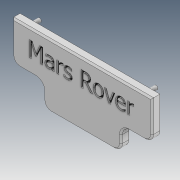
# Autodesk Inventor part: tampa parte de traz mars
Saved by Autodesk Inventor 2021 (Build 250183000, 183)
## iProperties
Created: 2020-11-19
Part Number: tampa parte de traz mars
Material: Genérico
Document SubType Name: Modeling
Designer: evert
Density: 1 g/cm^3
Appearance: Padrão
Author: evert
Autodesk Inventor part; units mm, degrees
ref_plane "YZ Plane" through (0, 0, 0) normal (1, 0, 0) x (0, 1, 0)
ref_plane "XZ Plane" through (0, 0, 0) normal (0, 1, 0) x (-1, 0, 0)
ref_plane "XY Plane" through (0, 0, 0) normal (0, 0, 1) x (1, 0, 0)
sketch "Esboço1" plane through (0, 0, 0) normal (0, 0, 1) x (1, 0, 0)
  line L0 (0, 0) -> (180, 0)
  line L1 (180, 0) -> (180, -50.8)
  line L2 (180, -50.8) -> (0, -50.8)
  line L3 (0, -50.8) -> (0, 0)
  line L4 (0, -50.8) -> (40, -50.8)
  line L5 (40, -50.8) -> (40, -80.8)
  line L6 (40, -80.8) -> (140, -80.8)
  line L7 (140, -80.8) -> (140, -50.8)
  dimension "d0" = 180
  dimension "d1" = 50.8
  dimension "d2" = 40
  dimension "d3" = 30
  dimension "d4" = 100
  constraints: 16 end point, 5 perpendicular, 2 point on line, 1 horizontal, 1 vertical
  measures "d0" distance of L0.start L0.end
  measures "d1" distance of L0.end L1.end
  measures "d2" distance of L2.end L4.end
  measures "d3" distance of L4.end L5.end
  measures "d4" distance of L5.end L6.end
extrude "Extrusão1" add sketch "Esboço1" along normal blind 10
sketch "Esboço3" plane through (0, 0, 0) normal (0, 0, -1) x (-1, 0, 0)
  line L0 (-40, -50.8) -> (-40, -80.8) projected
  line L1 (-40, -80.8) -> (0, -80.8) projected
  line L2 (-40, -50.8) -> (0, -50.8)
  line L3 (0, -50.8) -> (0, -80.8)
  line L4 (0, -80.8) -> (-40, -80.8)
  line L5 (-40, -80.8) -> (-40, -50.8)
  line L6 (-140, -50.8) -> (-180, -50.8) projected
  line L7 (-180, -40.4) -> (-180, -80.8) projected
  line L8 (-140, -50.8) -> (-180, -50.8)
  line L9 (-180, -50.8) -> (-180, -80.8)
  line L10 (-180, -80.8) -> (-140, -80.8)
  line L11 (-140, -80.8) -> (-140, -50.8)
  point P0 (0, 0)
  constraints: 16 end point, 4 parallel, 2 horizontal, 2 perpendicular
extrude "Extrusão3" cut sketch "Esboço3" against normal blind 180
sketch "Esboço4" plane through (0, 0, 0) normal (0, 0, -1) x (-1, 0, 0)
  line L0 (-180, 0) -> (0, 0) projected
  line L1 (0, 0) -> (-15, 0)
  line L2 (-15, 0) -> (-15, -5)
  line L3 (0, -8.08) -> (-180, -8.08) projected
  circle A0 centre (-15, -5) radius 2.5
  line L4 (0, -50.8) -> (0, -40.4) projected
  line L5 (0, -50.8) -> (-15, -50.8)
  line L6 (-15, -50.8) -> (-15, -35.8)
  circle A1 centre (-15, -35.8) radius 2.5
  line L7 (-40, -80.8) -> (-140, -80.8) projected
  line L8 (-40, -80.8) -> (-55, -80.8)
  line L9 (-55, -80.8) -> (-55, -65.8)
  circle A2 centre (-55, -65.8) radius 2.5
  line L10 (-140, -80.8) -> (-140, -50.8) projected
  line L11 (-140, -80.8) -> (-125, -80.8)
  line L12 (-125, -80.8) -> (-125, -65.8)
  circle A3 centre (-125, -65.8) radius 2.5
  line L13 (-140, -50.8) -> (-180, -50.8) projected
  line L14 (-180, -50.8) -> (-165, -50.8)
  line L15 (-165, -50.8) -> (-165, -35.8)
  circle A4 centre (-165, -35.8) radius 2.5
  line L16 (-180, 0) -> (-165, 0)
  line L17 (-165, 0) -> (-165, -5)
  circle A5 centre (-165, -5) radius 2.5
  dimension "d13" = 15
  dimension "d14" = 5
  dimension "d15" = 15
  dimension "d16" = 5
  dimension "d17" = 15
  dimension "d18" = 15
  dimension "d19" = 5
  dimension "d20" = 15
  dimension "d21" = 15
  dimension "d22" = 15
  constraints: 24 end point, 6 centre point, 6 coincident, 5 point on line, 4 perpendicular, 3 vertical
  measures "d13" distance of L0.end L1.end
  measures "d14" distance of L1.end L2.end
  measures "d15" distance of L5.end L6.end
  measures "d16" diameter of A1
  measures "d17" distance of L7.start L8.end
  measures "d18" distance of L8.end L9.end
  measures "d19" diameter of A2
  measures "d20" distance of L7.end L11.end
  measures "d21" distance of L11.end L12.end
  measures "d22" distance of L13.end L14.end
extrude "Extrusão4" add sketch "Esboço4" along normal blind 10
fillet "Arredondamento2" radius 10 6 edges at (140, -50.8, 5) (180, -50.8, 5) (140, -80.8, 5) (40, -80.8, 5) (40, -50.8, 5) (0, -50.8, 5)
chamfer "Chanfro1" distance 2 angle 45 6 edges at (90, 0, 10) (180, -20.4, 10) (0, -20.4, 10) (42.9289, -77.8711, 10) (90, -80.8, 10) (137.0711, -77.8711, 10)
sketch "Esboço7" plane through (0, 0, 10) normal (0, 0, 1) x (1, 0, 0)
  line L0 (20, -13.0888) -> (160, -13.0888) construction
  line L1 (160, -13.0888) -> (160, -33.5102) construction
  line L2 (160, -33.5102) -> (20, -33.5102) construction
  line L3 (20, -33.5102) -> (20, -13.0888) construction
  line L4 (2, -40.8) -> (2, -2) projected
  line L5 (178, -2) -> (178, -40.8) projected
  line L6 (39.1734, -33.0888) -> (36.5154, -33.0888)
  line L7 (36.5154, -33.0888) -> (36.5154, -15.8603)
  line L8 (36.5154, -15.8603) -> (31.2966, -27.5783)
  line L9 (31.2966, -27.5783) -> (29.6759, -27.5783)
  line L10 (29.6759, -27.5783) -> (24.5057, -15.8603)
  line L11 (24.5057, -15.8603) -> (24.5057, -33.0888)
  line L12 (24.5057, -33.0888) -> (22.0259, -33.0888)
  line L13 (22.0259, -33.0888) -> (22.0259, -13.0888)
  line L14 (22.0259, -13.0888) -> (25.6564, -13.0888)
  line L15 (25.6564, -13.0888) -> (30.6483, -24.2234)
  line L16 (30.6483, -24.2234) -> (35.4781, -13.0888)
  line L17 (35.4781, -13.0888) -> (39.1734, -13.0888)
  line L18 (39.1734, -13.0888) -> (39.1734, -33.0888)
  spline S0 degree 2 poles (51.3938, -31.5005) (51.0859, -31.7274) (50.0486, -32.5378) (49.5624, -32.7809) knots 0 0 0 1 2 2 2
  spline S1 degree 2 poles (49.5624, -32.7809) (48.8979, -33.1375) (47.6499, -33.5102) (46.5154, -33.5102) knots 0 0 0 1 2 2 2
  spline S2 degree 2 poles (46.5154, -33.5102) (45.5916, -33.5102) (43.9222, -32.8133) (43.2901, -32.1812) knots 0 0 0 1 2 2 2
  spline S3 degree 2 poles (43.2901, -32.1812) (42.6904, -31.5653) (41.9611, -29.7501) (41.9611, -28.7452) knots 0 0 0 1 2 2 2
  spline S4 degree 2 poles (41.9611, -28.7452) (41.9611, -27.1893) (43.2739, -24.9851) (44.7002, -24.353) knots 0 0 0 1 2 2 2
  spline S5 degree 2 poles (44.7002, -24.353) (45.9643, -23.7696) (49.4003, -23.332) (51.3938, -23.2185) knots 0 0 0 1 2 2 2
  line L19 (51.3938, -23.2185) -> (51.3938, -22.7323)
  spline S6 degree 2 poles (51.3938, -22.7323) (51.3938, -21.8571) (50.859, -20.7712) (50.3728, -20.4632) knots 0 0 0 1 2 2 2
  spline S7 degree 2 poles (50.3728, -20.4632) (49.8865, -20.1553) (48.4927, -19.9608) (47.7472, -19.9608) knots 0 0 0 1 2 2 2
  spline S8 degree 2 poles (47.7472, -19.9608) (46.872, -19.9608) (44.5057, -20.4794) (43.3225, -20.9819) knots 0 0 0 1 2 2 2
  line L20 (43.3225, -20.9819) -> (43.1767, -20.9819)
  line L21 (43.1767, -20.9819) -> (43.1767, -18.4049)
  spline S9 degree 2 poles (43.1767, -18.4049) (43.8736, -18.2104) (46.483, -17.7242) (47.7634, -17.7242) knots 0 0 0 1 2 2 2
  spline S10 degree 2 poles (47.7634, -17.7242) (49.3193, -17.7242) (51.4425, -18.2104) (52.2853, -18.8425) knots 0 0 0 1 2 2 2
  spline S11 degree 2 poles (52.2853, -18.8425) (53.1118, -19.4584) (53.9222, -21.4195) (53.9222, -22.8295) knots 0 0 0 1 2 2 2
  line L22 (53.9222, -22.8295) -> (53.9222, -33.0888)
  line L23 (53.9222, -33.0888) -> (51.3938, -33.0888)
  line L24 (51.3938, -33.0888) -> (51.3938, -31.5005)
  line L25 (51.3938, -29.3935) -> (51.3938, -25.2282)
  spline S12 degree 2 poles (51.3938, -25.2282) (50.4862, -25.3093) (47.7472, -25.5848) (46.8882, -25.8441) knots 0 0 0 1 2 2 2
  spline S13 degree 2 poles (46.8882, -25.8441) (45.8833, -26.1521) (44.5705, -27.4324) (44.5705, -28.567) knots 0 0 0 1 2 2 2
  spline S14 degree 2 poles (44.5705, -28.567) (44.5705, -29.8636) (46.0292, -31.1764) (47.423, -31.1764) knots 0 0 0 1 2 2 2
  spline S15 degree 2 poles (47.423, -31.1764) (48.6062, -31.1764) (50.5511, -30.1553) (51.3938, -29.3935) knots 0 0 0 1 2 2 2
  line L26 (65.4295, -20.7874) -> (65.2998, -20.7874)
  spline S16 degree 2 poles (65.2998, -20.7874) (65.0081, -20.7063) (64.376, -20.6739) (63.9384, -20.6739) knots 0 0 0 1 2 2 2
  spline S17 degree 2 poles (63.9384, -20.6739) (62.9173, -20.6739) (60.9076, -21.5653) (60, -22.4405) knots 0 0 0 1 2 2 2
  line L27 (60, -22.4405) -> (60, -33.0888)
  line L28 (60, -33.0888) -> (57.4716, -33.0888)
  line L29 (57.4716, -33.0888) -> (57.4716, -18.0807)
  line L30 (57.4716, -18.0807) -> (60, -18.0807)
  line L31 (60, -18.0807) -> (60, -20.3174)
  spline S18 degree 2 poles (60, -20.3174) (61.3776, -19.0856) (63.436, -18.0807) (64.4084, -18.0807) knots 0 0 0 1 2 2 2
  spline S19 degree 2 poles (64.4084, -18.0807) (64.7974, -18.0807) (65.1864, -18.1132) (65.4295, -18.1618) knots 0 0 0 1 2 2 2
  line L32 (65.4295, -18.1618) -> (65.4295, -20.7874)
  spline S20 degree 2 poles (71.4425, -33.4454) (69.9352, -33.4454) (67.3258, -32.635) (66.4668, -32.1812) knots 0 0 0 1 2 2 2
  line L33 (66.4668, -32.1812) -> (66.4668, -29.3449)
  line L34 (66.4668, -29.3449) -> (66.5964, -29.3449)
  spline S21 degree 2 poles (66.5964, -29.3449) (66.9206, -29.6042) (67.7958, -30.2201) (68.5251, -30.5605) knots 0 0 0 1 2 2 2
  spline S22 degree 2 poles (68.5251, -30.5605) (69.1572, -30.8684) (70.7131, -31.3222) (71.5397, -31.3222) knots 0 0 0 1 2 2 2
  spline S23 degree 2 poles (71.5397, -31.3222) (72.1394, -31.3222) (73.517, -31.0467) (73.8412, -30.8198) knots 0 0 0 1 2 2 2
  spline S24 degree 2 poles (73.8412, -30.8198) (74.3112, -30.5119) (74.7326, -29.8149) (74.7326, -29.1018) knots 0 0 0 1 2 2 2
  spline S25 degree 2 poles (74.7326, -29.1018) (74.7326, -28.2104) (73.7601, -27.2866) (72.5122, -26.9786) knots 0 0 0 1 2 2 2
  spline S26 degree 2 poles (72.5122, -26.9786) (72.0259, -26.8652) (70.47, -26.541) (69.8055, -26.3627) knots 0 0 0 1 2 2 2
  spline S27 degree 2 poles (69.8055, -26.3627) (68.0875, -25.8603) (66.5316, -23.7858) (66.5316, -22.3109) knots 0 0 0 1 2 2 2
  spline S28 degree 2 poles (66.5316, -22.3109) (66.5316, -20.2687) (69.5948, -17.7242) (72.1232, -17.7242) knots 0 0 0 1 2 2 2
  spline S29 degree 2 poles (72.1232, -17.7242) (73.3712, -17.7242) (75.8995, -18.3401) (76.7585, -18.8101) knots 0 0 0 1 2 2 2
  line L35 (76.7585, -18.8101) -> (76.7585, -21.5167)
  line L36 (76.7585, -21.5167) -> (76.6288, -21.5167)
  spline S30 degree 2 poles (76.6288, -21.5167) (75.6564, -20.7388) (73.2901, -19.8474) (72.0746, -19.8474) knots 0 0 0 1 2 2 2
  spline S31 degree 2 poles (72.0746, -19.8474) (70.8266, -19.8474) (69.1086, -20.9008) (69.1086, -21.9543) knots 0 0 0 1 2 2 2
  spline S32 degree 2 poles (69.1086, -21.9543) (69.1086, -22.9106) (70.1297, -23.8344) (71.2642, -24.1261) knots 0 0 0 1 2 2 2
  spline S33 degree 2 poles (71.2642, -24.1261) (71.8152, -24.272) (73.2091, -24.5637) (73.9708, -24.742) knots 0 0 0 1 2 2 2
  spline S34 degree 2 poles (73.9708, -24.742) (75.624, -25.1634) (77.3096, -27.0921) (77.3096, -28.7615) knots 0 0 0 1 2 2 2
  spline S35 degree 2 poles (77.3096, -28.7615) (77.3096, -29.7339) (76.5478, -31.4519) (75.8023, -32.084) knots 0 0 0 1 2 2 2
  spline S36 degree 2 poles (75.8023, -32.084) (75.0081, -32.7485) (72.9822, -33.4454) (71.4425, -33.4454) knots 0 0 0 1 2 2 2
  line L37 (103.9222, -33.0888) -> (100.47, -33.0888)
  line L38 (100.47, -33.0888) -> (94.1491, -25.131)
  line L39 (94.1491, -25.131) -> (91.1021, -25.131)
  line L40 (91.1021, -25.131) -> (91.1021, -33.0888)
  line L41 (91.1021, -33.0888) -> (88.4441, -33.0888)
  line L42 (88.4441, -33.0888) -> (88.4441, -13.0888)
  line L43 (88.4441, -13.0888) -> (93.5981, -13.0888)
  spline S37 degree 2 poles (93.5981, -13.0888) (95.316, -13.0888) (97.6337, -13.4616) (98.6872, -14.1423) knots 0 0 0 1 2 2 2
  spline S38 degree 2 poles (98.6872, -14.1423) (99.7407, -14.823) (100.9562, -16.9462) (100.9562, -18.5183) knots 0 0 0 1 2 2 2
  spline S39 degree 2 poles (100.9562, -18.5183) (100.9562, -20.7063) (98.7196, -23.6723) (96.8071, -24.3854) knots 0 0 0 1 2 2 2
  line L44 (96.8071, -24.3854) -> (103.9222, -33.0888)
  spline S40 degree 2 poles (98.1848, -18.729) (98.1848, -17.8538) (97.5689, -16.5086) (96.9206, -16.071) knots 0 0 0 1 2 2 2
  spline S41 degree 2 poles (96.9206, -16.071) (96.3533, -15.6982) (94.846, -15.3903) (93.7439, -15.3903) knots 0 0 0 1 2 2 2
  line L45 (93.7439, -15.3903) -> (91.1021, -15.3903)
  line L46 (91.1021, -15.3903) -> (91.1021, -22.9106)
  line L47 (91.1021, -22.9106) -> (93.436, -22.9106)
  spline S42 degree 2 poles (93.436, -22.9106) (94.5867, -22.9106) (96.4182, -22.5054) (97.0502, -21.8733) knots 0 0 0 1 2 2 2
  spline S43 degree 2 poles (97.0502, -21.8733) (97.6337, -21.3222) (98.1848, -19.7663) (98.1848, -18.729) knots 0 0 0 1 2 2 2
  spline S44 degree 2 poles (117.6499, -25.5848) (117.6499, -29.3773) (114.0032, -33.5102) (110.9562, -33.5102) knots 0 0 0 1 2 2 2
  spline S45 degree 2 poles (110.9562, -33.5102) (107.8282, -33.5102) (104.2464, -29.2477) (104.2464, -25.5848) knots 0 0 0 1 2 2 2
  spline S46 degree 2 poles (104.2464, -25.5848) (104.2464, -21.8247) (107.9417, -17.6593) (110.9562, -17.6593) knots 0 0 0 1 2 2 2
  spline S47 degree 2 poles (110.9562, -17.6593) (114.0032, -17.6593) (117.6499, -21.8085) (117.6499, -25.5848) knots 0 0 0 1 2 2 2
  spline S48 degree 2 poles (115.0405, -25.5848) (115.0405, -22.6674) (112.9173, -19.8311) (110.9562, -19.8311) knots 0 0 0 1 2 2 2
  spline S49 degree 2 poles (110.9562, -19.8311) (108.9951, -19.8311) (106.8558, -22.6674) (106.8558, -25.5848) knots 0 0 0 1 2 2 2
  spline S50 degree 2 poles (106.8558, -25.5848) (106.8558, -28.4211) (108.9951, -31.3384) (110.9562, -31.3384) knots 0 0 0 1 2 2 2
  spline S51 degree 2 poles (110.9562, -31.3384) (112.9011, -31.3384) (115.0405, -28.4697) (115.0405, -25.5848) knots 0 0 0 1 2 2 2
  line L48 (132.0259, -18.0807) -> (126.3695, -33.0888)
  line L49 (126.3695, -33.0888) -> (124.1005, -33.0888)
  line L50 (124.1005, -33.0888) -> (118.4927, -18.0807)
  line L51 (118.4927, -18.0807) -> (121.2318, -18.0807)
  line L52 (121.2318, -18.0807) -> (125.3323, -29.6367)
  line L53 (125.3323, -29.6367) -> (129.4003, -18.0807)
  line L54 (129.4003, -18.0807) -> (132.0259, -18.0807)
  spline S52 degree 2 poles (140.4538, -33.4292) (136.8558, -33.4292) (132.9011, -29.3935) (132.9011, -25.6658) knots 0 0 0 1 2 2 2
  spline S53 degree 2 poles (132.9011, -25.6658) (132.9011, -22.0029) (136.7423, -17.6593) (139.8379, -17.6593) knots 0 0 0 1 2 2 2
  spline S54 degree 2 poles (139.8379, -17.6593) (141.2318, -17.6593) (143.3874, -18.4697) (144.1815, -19.3287) knots 0 0 0 1 2 2 2
  spline S55 degree 2 poles (144.1815, -19.3287) (144.9919, -20.1877) (145.8509, -22.6674) (145.8509, -24.4665) knots 0 0 0 1 2 2 2
  line L55 (145.8509, -24.4665) -> (145.8509, -25.8441)
  line L56 (145.8509, -25.8441) -> (135.4619, -25.8441)
  spline S56 degree 2 poles (135.4619, -25.8441) (135.4619, -28.4535) (138.0875, -31.225) (140.4214, -31.225) knots 0 0 0 1 2 2 2
  spline S57 degree 2 poles (140.4214, -31.225) (141.248, -31.225) (142.8525, -30.8522) (143.5008, -30.5605) knots 0 0 0 1 2 2 2
  spline S58 degree 2 poles (143.5008, -30.5605) (144.1815, -30.2363) (145.1216, -29.6691) (145.4295, -29.4097) knots 0 0 0 1 2 2 2
  line L57 (145.4295, -29.4097) -> (145.5754, -29.4097)
  line L58 (145.5754, -29.4097) -> (145.5754, -32.165)
  spline S59 degree 2 poles (145.5754, -32.165) (145.1378, -32.3433) (143.8088, -32.8619) (143.2901, -33.0078) knots 0 0 0 1 2 2 2
  spline S60 degree 2 poles (143.2901, -33.0078) (142.5608, -33.2185) (141.3614, -33.4292) (140.4538, -33.4292) knots 0 0 0 1 2 2 2
  spline S61 degree 2 poles (143.3874, -23.9154) (143.3549, -22.8944) (142.9335, -21.4033) (142.5284, -20.9008) knots 0 0 0 1 2 2 2
  spline S62 degree 2 poles (142.5284, -20.9008) (142.0908, -20.3336) (140.7131, -19.7339) (139.6921, -19.7339) knots 0 0 0 1 2 2 2
  spline S63 degree 2 poles (139.6921, -19.7339) (138.6872, -19.7339) (137.2771, -20.3336) (136.6937, -20.917) knots 0 0 0 1 2 2 2
  spline S64 degree 2 poles (136.6937, -20.917) (136.1264, -21.5167) (135.5429, -22.9592) (135.4619, -23.9154) knots 0 0 0 1 2 2 2
  line L59 (135.4619, -23.9154) -> (143.3874, -23.9154)
  line L60 (156.3695, -20.7874) -> (156.2399, -20.7874)
  spline S65 degree 2 poles (156.2399, -20.7874) (155.9481, -20.7063) (155.316, -20.6739) (154.8784, -20.6739) knots 0 0 0 1 2 2 2
  spline S66 degree 2 poles (154.8784, -20.6739) (153.8574, -20.6739) (151.8476, -21.5653) (150.94, -22.4405) knots 0 0 0 1 2 2 2
  line L61 (150.94, -22.4405) -> (150.94, -33.0888)
  line L62 (150.94, -33.0888) -> (148.4117, -33.0888)
  line L63 (148.4117, -33.0888) -> (148.4117, -18.0807)
  line L64 (148.4117, -18.0807) -> (150.94, -18.0807)
  line L65 (150.94, -18.0807) -> (150.94, -20.3174)
  spline S67 degree 2 poles (150.94, -20.3174) (152.3177, -19.0856) (154.376, -18.0807) (155.3485, -18.0807) knots 0 0 0 1 2 2 2
  spline S68 degree 2 poles (155.3485, -18.0807) (155.7374, -18.0807) (156.1264, -18.1132) (156.3695, -18.1618) knots 0 0 0 1 2 2 2
  line L66 (156.3695, -18.1618) -> (156.3695, -20.7874)
  point P0 (0, 0)
  dimension "d33" = 18
  dimension "d34" = 18
  constraints: 2 other
  measures "d33" distance between parallel lines of L4 L3
  measures "d34" distance between parallel lines of L5 L1
extrude "Extrusão6" cut sketch "Esboço7" against normal blind 2
